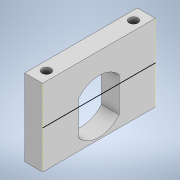
# Autodesk Inventor part: motor_back
Saved by Autodesk Inventor 2020 (Build 240168000, 168)
## iProperties
Created: 2023-11-06
Part Number: motor_back
Material: Типовые
Document SubType Name: Modeling
Designer: denis
Density: 1 g/cm^3
Appearance: По умолчанию
Author: denis
Autodesk Inventor part; units mm, degrees
ref_plane "YZ Plane" through (0, 0, 0) normal (1, 0, 0) x (0, 1, 0)
ref_plane "XZ Plane" through (0, 0, 0) normal (0, 1, 0) x (-1, 0, 0)
ref_plane "XY Plane" through (0, 0, 0) normal (0, 0, 1) x (1, 0, 0)
sketch "Эскиз1" plane through (0, 0, 0) normal (0, 1, 0) x (-1, 0, 0)
  line L0 (7, 44) -> (0, 44)
  line L1 (0, 44) -> (0, 0)
  line L2 (0, 0) -> (7, 0)
  line L3 (7, 0) -> (7, 44)
  circle A0 centre (3.5, 39) radius 1.75
  line L4 (3.5, 44) -> (3.5, 0) construction
  line L5 (7, 22) -> (0, 22) construction
  circle A1 centre (3.5, 5) radius 1.75
  line L6 (0, 0) -> (21.6964, 0) construction
  line L7 (0, 0) -> (0, 52.547) construction
  point P0 (14.925, 0)
  point P1 (0, 24.3748)
  dimension "d0" = 44
  dimension "d1" = 7
  dimension "d2" = 3.5
  dimension "d3" = 34
  constraints: 16 end point, 3 horizontal, 3 perpendicular, 2 centre point, 2 collinear, 2 midpoint, 2 parallel, 2 vertical, 1 point on line, 1 symmetric about line, 1 other
  measures "d0" distance of L2.end L0.start
  measures "d1" distance of L0.start L0.end
  measures "d2" diameter of A0
  measures "d3" distance of A1.centre A0.centre
extrude "Выдавливание1" add sketch "Эскиз1" along normal blind 30
sketch "Эскиз2" plane through (0, 0, 44) normal (1, 0, 0) x (0, 0, -1)
  line L0 (0, 0) -> (44, 0) construction
  line L1 (44, 0) -> (44, 30) construction
  line L2 (0, 30) -> (44, 30) construction
  line L3 (0, 0) -> (0, 30) construction
  line L4 (0, 30) -> (44, 30) construction
  line L5 (22, 30) -> (22, 0) construction
  line L6 (0, 0) -> (0, 30) construction
  line L7 (0, 15) -> (44, 15) construction
  line L8 (44, 0) -> (44, 30) construction
  arc A0 (14.05, 17.9823) -> (14.05, 4.4177) centre (22, 11.2) ccw construction
  line L9 (14.05, 17.9823) -> (14.05, 4.4177)
  line L10 (29.95, 17.9823) -> (29.95, 4.4177)
  arc A1 (22, 21.65) -> (14.05, 17.9823) centre (22, 11.2) ccw
  arc A2 (29.95, 17.9823) -> (22, 21.65) centre (22, 11.2) ccw
  arc A3 (29.95, 4.4177) -> (29.95, 17.9823) centre (22, 11.2) ccw construction
  arc A4 (22, 0.75) -> (29.95, 4.4177) centre (22, 11.2) ccw
  arc A5 (14.05, 4.4177) -> (22, 0.75) centre (22, 11.2) ccw
  dimension "d6" = 11.2
  dimension "d7" = 20.9
  dimension "d8" = 15.9
  constraints: 15 point on circle, 8 end point, 6 centre point, 4 midpoint, 3 point on line, 2 symmetric about line, 1 coincident, 1 vertical
  measures "d6" distance from line of L0 point (22, 11.2)
  measures "d7" diameter of A0
  measures "d8" distance between parallel lines of L10 L9
extrude "Выдавливание2" cut sketch "Эскиз2" against normal blind 30
sketch "Эскиз3" plane through (0, 0, 44) normal (1, 0, 0) x (0, 0, -1)
  line L0 (44, 0) -> (44, 30) construction
  line L1 (0, 0) -> (0, 30) construction
  line L2 (0, 0) -> (0, 30) construction
  line L3 (0, 15) -> (44, 15)
  constraints: 2 end point, 2 midpoint
